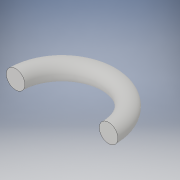
# Autodesk Inventor part: Tube
Saved by Autodesk Inventor 2017 (Build 210142000, 142)
## iProperties
Created: 2016-09-15
Part Number: Tube
Material: Generic
Document SubType Name: Modeling
Designer: Spartacles
Density: 1 g/cm^3
Appearance: Default
Author: Spartacles
Autodesk Inventor part; units mm, degrees
ref_plane "YZ Plane" through (0, 0, 0) normal (1, 0, 0) x (0, 1, 0)
ref_plane "XZ Plane" through (0, 0, 0) normal (0, 1, 0) x (-1, 0, 0)
ref_plane "XY Plane" through (0, 0, 0) normal (0, 0, 1) x (1, 0, 0)
sketch "Sketch3" plane through (0, 0, 0) normal (0, 0, 1) x (1, 0, 0)
  circle A0 centre (0, 0) radius 38.1
  circle A1 centre (381, 0) radius 38.1
  dimension "d2" = 76.2
  dimension "d3" = 76.2
  dimension "d4" = 381
  constraints: 2 centre point
  measures "d2" diameter of A0
  measures "d3" diameter of A1
  measures "d4" distance of A1.centre point (0, 0)
sketch "Sketch4" plane through (0, 0, 0) normal (0, 1, 0) x (-1, 0, 0)
  arc A0 (-381, 0) -> (0, 0) centre (-190.5, 0) ccw
  line L0 (0, 0) -> (-381, 0) construction
  dimension "d6" = 381
  constraints: 2 end point, 2 point on circle, 1 centre point, 1 horizontal
  measures "d6" diameter of A0
sweep "Sweep1" add profiles "Sketch3" path "Sketch4"
equation "\"d3\" = d2"
body "Solid1"
